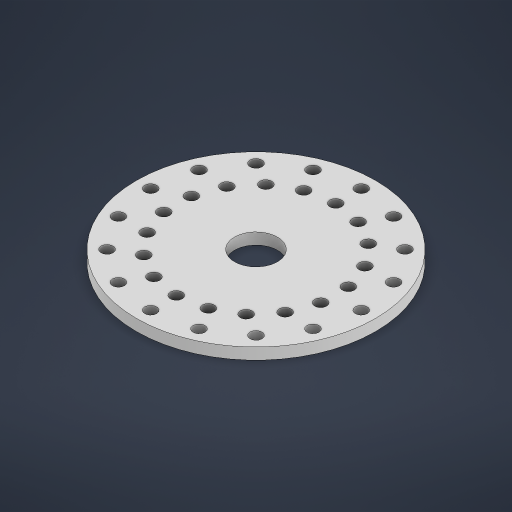
# Autodesk Inventor part: HousingFaceMount
Saved by Autodesk Inventor 2024 (Build 280153000, 153)
## iProperties
Created: 2024-03-11
Part Number: HousingFaceMount
Material: Generic
Document SubType Name: Modeling
Designer: avsar
Density: 1 g/cm^3
Appearance: Default
Author: avsar
Autodesk Inventor part; units mm, degrees
ref_plane "YZ Plane" through (0, 0, 0) normal (1, 0, 0) x (0, 1, 0)
ref_plane "XZ Plane" through (0, 0, 0) normal (0, 1, 0) x (-1, 0, 0)
ref_plane "XY Plane" through (0, 0, 0) normal (0, 0, 1) x (1, 0, 0)
sketch "Sketch1" plane through (0, 0, 0) normal (0, 1, 0) x (-1, 0, 0)
  circle A0 centre (0, 0) radius 42
  circle A1 centre (0, -28) radius 2.1
  circle A2 centre (0, -28) radius 4.1 construction
  circle A3 centre (9.5766, -26.3114) radius 2.1
  circle A4 centre (17.9981, -21.4492) radius 2.1
  circle A5 centre (24.2487, -14) radius 2.1
  circle A6 centre (27.5746, -4.8621) radius 2.1
  circle A7 centre (27.5746, 4.8621) radius 2.1
  circle A8 centre (24.2487, 14) radius 2.1
  circle A9 centre (17.9981, 21.4492) radius 2.1
  circle A10 centre (9.5766, 26.3114) radius 2.1
  circle A11 centre (0, 28) radius 2.1
  circle A12 centre (-9.5766, 26.3114) radius 2.1
  circle A13 centre (-17.9981, 21.4492) radius 2.1
  circle A14 centre (-24.2487, 14) radius 2.1
  circle A15 centre (-27.5746, 4.8621) radius 2.1
  circle A16 centre (-27.5746, -4.8621) radius 2.1
  circle A17 centre (-24.2487, -14) radius 2.1
  circle A18 centre (-17.9981, -21.4492) radius 2.1
  circle A19 centre (-9.5766, -26.3114) radius 2.1
  circle A20 centre (0, 0) radius 7.55
  circle A21 centre (9.5766, -26.3114) radius 4.1 construction
  circle A22 centre (0, -37) radius 2.1
  circle A23 centre (0, -37) radius 4 construction
  circle A24 centre (14.1593, -34.1835) radius 2.1
  circle A25 centre (26.163, -26.163) radius 2.1
  circle A26 centre (34.1835, -14.1593) radius 2.1
  circle A27 centre (37, 0) radius 2.1
  circle A28 centre (34.1835, 14.1593) radius 2.1
  circle A29 centre (26.163, 26.163) radius 2.1
  circle A30 centre (14.1593, 34.1835) radius 2.1
  circle A31 centre (0, 37) radius 2.1
  circle A32 centre (-14.1593, 34.1835) radius 2.1
  circle A33 centre (-26.163, 26.163) radius 2.1
  circle A34 centre (-34.1835, 14.1593) radius 2.1
  circle A35 centre (-37, 0) radius 2.1
  circle A36 centre (-34.1835, -14.1593) radius 2.1
  circle A37 centre (-26.163, -26.163) radius 2.1
  circle A38 centre (-14.1593, -34.1835) radius 2.1
  dimension "d4" = 84
  dimension "d5" = 4.2
  dimension "d6" = 28
  dimension "d7" = 8.2
  dimension "d8" = 360
  dimension "d9" = 15.1
  dimension "d10" = 8.2
  dimension "d11" = 4.2
  dimension "d12" = 37
  dimension "d13" = 8
  dimension "d14" = 360
  constraints: 39 centre point, 6 coincident, 2 vertical alignment, 70 other
  measures "d4" diameter of A0
  measures "d5" diameter of A1
  measures "d6" distance of point (0, 0) A1.centre
  measures "d7" diameter of A2
  measures "d9" diameter of A20
  measures "d10" diameter of A21
  measures "d11" diameter of A22
  measures "d12" distance of point (0, 0) A22.centre
  measures "d13" diameter of A23
extrude "Extrusion1" add sketch "Sketch1" along normal blind 4
body "Solid1"
